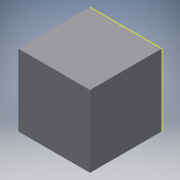
# Autodesk Inventor part: Heat Sink v2
Saved by Autodesk Inventor 2019 Beta2 (Build 230110000, 110) ContinuousBuild 0
## iProperties
Created: 2012-08-29
Part Number: Heat Sink v2
Material: Generic
Document SubType Name: Modeling
Designer: John
Density: 1 g/cm^3
Appearance: Default
Author: John
Autodesk Inventor part; units mm, degrees
ref_plane "YZ Plane" through (0, 0, 0) normal (1, 0, 0) x (0, 1, 0)
ref_plane "XZ Plane" through (0, 0, 0) normal (0, 1, 0) x (-1, 0, 0)
ref_plane "XY Plane" through (0, 0, 0) normal (0, 0, 1) x (1, 0, 0)
sketch "Sketch1" plane through (0, 0, 0) normal (0, 0, 1) x (1, 0, 0)
  line L0 (-20.0025, -20.0025) -> (20.0025, -20.0025)
  line L1 (20.0025, -20.0025) -> (20.0025, 20.0025)
  line L2 (20.0025, 20.0025) -> (-20.0025, 20.0025)
  line L3 (-20.0025, 20.0025) -> (-20.0025, -20.0025)
  line L4 (-20.0025, -20.0025) -> (20.0025, 20.0025) construction
  line L5 (20.0025, -20.0025) -> (-20.0025, 20.0025) construction
  point P0 (0, 0)
  dimension "d0" = 40.005
  dimension "d1" = 40.005
  constraints: 12 end point, 2 midpoint, 2 parallel, 1 horizontal, 1 perpendicular
  measures "d0" distance of L2.end L1.end
  measures "d1" distance of L1.end L0.end
extrude "Extrusion1" add sketch "Sketch1" along normal blind 40.005
sketch "Sketch2" plane through (0, 0, 0) normal (0, 0, -1) x (-1, 0, 0)
  line L0 (20.0025, -20.0025) -> (-20.0025, -20.0025) projected
  line L1 (20.0025, 20.0025) -> (20.0025, -20.0025) projected
  line L2 (-20.0025, 20.0025) -> (20.0025, 20.0025) projected
  line L3 (-20.0025, -20.0025) -> (-20.0025, 20.0025) projected
  point P0 (0, 0)
body "Solid1"
